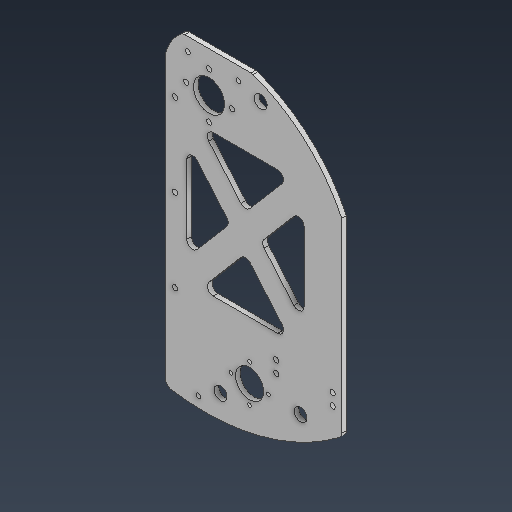
# Autodesk Inventor part: стенка пуляло
Saved by Autodesk Inventor 2026 (Build 300175000, 175)
## iProperties
Created: 2025-11-22
Part Number: стенка пуляло
Material: Типовые
Document SubType Name: Modeling
Designer: Phantom
Density: 1 g/cm^3
Appearance: По умолчанию
Author: Phantom
Autodesk Inventor part; units mm, degrees
(part 1 of 2)
ref_plane "YZ Plane" through (0, 0, 0) normal (1, 0, 0) x (0, 1, 0)
ref_plane "XZ Plane" through (0, 0, 0) normal (0, 1, 0) x (-1, 0, 0)
ref_plane "XY Plane" through (0, 0, 0) normal (0, 0, 1) x (1, 0, 0)
sketch "Эскиз1" plane through (0, 0, 0) normal (0, 0, 1) x (1, 0, 0)
  line L0 (0, 0) -> (150, 0)
  line L1 (150, 0) -> (150, 380)
  line L2 (150, 380) -> (0, 380)
  line L3 (0, 380) -> (0, 0)
  dimension "d2" = 150
  dimension "d3" = 380
  constraints: 8 end point, 2 parallel, 1 horizontal, 1 perpendicular
  measures "d2" distance of L1.end L2.end
  measures "d3" distance of L2.end L0.start
extrude "Выдавливание1" add sketch "Эскиз1" along normal blind 4
sketch "Эскиз3" plane through (0, 0, 0) normal (0, 0, -1) x (-1, 0, 0)
  circle A0 centre (-37, 259.345) radius 3.25
  line L0 (-150, 380) -> (0, 380) projected
  line L1 (0, 380) -> (0, 0) projected
  circle A1 centre (-37, 259.345) radius 203.5
  circle A2 centre (-71.5472, 58.7989) radius 12
  circle A3 centre (-63.3281, 72.5265) radius 1.6
  circle A4 centre (-55.5492, 58.5447) radius 1.6
  circle A5 centre (-63.7683, 44.8172) radius 1.6
  circle A6 centre (-79.7662, 45.0713) radius 1.6
  circle A7 centre (-87.5451, 59.053) radius 1.6
  circle A8 centre (-79.3261, 72.7806) radius 1.6
  line L2 (-162.8639, 128.9118) -> (-165.6991, 126.0733) projected
  arc A9 (-165.6991, 126.0733) -> (-166.6166, 122.0185) centre (-139.5582, 118.0273) ccw projected
  arc A10 (-166.6166, 122.0185) -> (-165.4337, 121.2858) centre (-47.0897, 313.6766) ccw projected
  arc A11 (-165.4337, 121.2858) -> (-162.2121, 123.9136) centre (-181.0608, 143.7331) ccw projected
  arc A12 (-162.2121, 123.9136) -> (-161.041, 123.208) centre (-47.0897, 313.6766) ccw projected
  arc A13 (-161.041, 123.208) -> (-161.8583, 119.1318) centre (-134.7098, 115.8085) ccw projected
  arc A14 (-161.8583, 119.1318) -> (-160.6577, 118.4286) centre (-47.0897, 313.6766) ccw projected
  arc A15 (-160.6577, 118.4286) -> (-157.5019, 121.1349) centre (-176.8332, 140.484) ccw projected
  arc A16 (-157.5019, 121.1349) -> (-156.3138, 120.4584) centre (-47.0897, 313.6766) ccw projected
  arc A17 (-156.3138, 120.4584) -> (-157.0304, 116.3633) centre (-129.8082, 113.7098) ccw projected
  arc A18 (-157.0304, 116.3633) -> (-155.8129, 115.6898) centre (-47.0897, 313.6766) ccw projected
  arc A19 (-155.8129, 115.6898) -> (-152.7247, 118.473) centre (-172.5268, 137.34) ccw projected
  arc A20 (-152.7247, 118.473) -> (-151.5202, 117.826) centre (-47.0897, 313.6766) ccw projected
  arc A21 (-151.5202, 117.826) -> (-152.1357, 113.7145) centre (-124.8564, 111.7326) ccw projected
  arc A22 (-152.1357, 113.7145) -> (-150.902, 113.0712) centre (-47.0897, 313.6766) ccw projected
  arc A23 (-150.902, 113.0712) -> (-147.8833, 115.9297) centre (-168.1442, 134.3031) ccw projected
  arc A24 (-147.8833, 115.9297) -> (-146.6632, 115.3126) centre (-47.0897, 313.6766) ccw projected
  arc A25 (-146.6632, 115.3126) -> (-147.1773, 111.1871) centre (-119.8574, 109.8779) ccw projected
  arc A26 (-147.1773, 111.1871) -> (-145.928, 110.5745) centre (-47.0897, 313.6766) ccw projected
  arc A27 (-145.928, 110.5745) -> (-142.9807, 113.5064) centre (-163.6882, 131.375) ccw projected
  arc A28 (-142.9807, 113.5064) -> (-141.7458, 112.9195) centre (-47.0897, 313.6766) ccw projected
  arc A29 (-141.7458, 112.9195) -> (-142.1581, 108.7827) centre (-114.8143, 108.1469) ccw projected
  arc A30 (-142.1581, 108.7827) -> (-140.8941, 108.201) centre (-47.0897, 313.6766) ccw projected
  arc A31 (-140.8941, 108.201) -> (-138.0199, 111.2047) centre (-159.1613, 128.5577) ccw projected
  arc A32 (-138.0199, 111.2047) -> (-136.771, 110.6484) centre (-47.0897, 313.6766) ccw projected
  arc A33 (-136.771, 110.6484) -> (-137.0811, 106.5027) centre (-109.73, 106.5408) ccw projected
  arc A34 (-137.0811, 106.5027) -> (-135.8033, 105.9522) centre (-47.0897, 313.6766) ccw projected
  arc A35 (-135.8033, 105.9522) -> (-133.0039, 109.0259) centre (-154.5665, 125.8527) ccw projected
  arc A36 (-133.0039, 109.0259) -> (-131.7416, 108.5005) centre (-47.0897, 313.6766) ccw projected
  arc A37 (-131.7416, 108.5005) -> (-131.9496, 104.3484) centre (-104.6077, 105.0603) ccw projected
  arc A38 (-131.9496, 104.3484) -> (-130.6585, 103.8296) centre (-47.0897, 313.6766) ccw projected
  arc A39 (-130.6585, 103.8296) -> (-127.9358, 106.9713) centre (-149.9063, 123.2618) ccw projected
  arc A40 (-127.9358, 106.9713) -> (-126.6609, 106.4772) centre (-47.0897, 313.6766) ccw projected
  arc A41 (-126.6609, 106.4772) -> (-126.7665, 102.3212) centre (-99.4504, 103.7066) ccw projected
  arc A42 (-126.7665, 102.3212) -> (-125.4631, 101.8344) centre (-47.0897, 313.6766) ccw projected
  arc A43 (-125.4631, 101.8344) -> (-122.8185, 105.0422) centre (-145.1838, 120.7864) ccw projected
  arc A44 (-122.8185, 105.0422) -> (-121.5319, 104.5796) centre (-47.0897, 313.6766) ccw projected
  arc A45 (-121.5319, 104.5796) -> (-121.5351, 100.4223) centre (-94.2614, 102.4803) ccw projected
  arc A46 (-121.5351, 100.4223) -> (-120.22, 99.9678) centre (-47.0897, 313.6766) ccw projected
  arc A47 (-120.22, 99.9678) -> (-117.6553, 103.2397) centre (-140.4017, 118.4282) ccw projected
  arc A48 (-117.6553, 103.2397) -> (-116.3577, 102.8091) centre (-47.0897, 313.6766) ccw projected
  arc A49 (-116.3577, 102.8091) -> (-116.2584, 98.6529) centre (-89.0438, 101.3822) ccw projected
  arc A50 (-116.2584, 98.6529) -> (-114.9326, 98.2309) centre (-47.0897, 313.6766) ccw projected
  arc A51 (-114.9326, 98.2309) -> (-112.4493, 101.5651) centre (-135.5629, 116.1885) ccw projected
  arc A52 (-112.4493, 101.5651) -> (-111.1414, 101.1665) centre (-47.0897, 313.6766) ccw projected
  arc A53 (-111.1414, 101.1665) -> (-110.9398, 97.014) centre (-83.8006, 100.413) ccw projected
  arc A54 (-110.9398, 97.014) -> (-109.604, 96.6248) centre (-47.0897, 313.6766) ccw projected
  arc A55 (-109.604, 96.6248) -> (-107.2035, 100.0192) centre (-130.6705, 114.0687) ccw projected
  arc A56 (-107.2035, 100.0192) -> (-105.8863, 99.6529) centre (-47.0897, 313.6766) ccw projected
  arc A57 (-105.8863, 99.6529) -> (-105.5824, 95.5067) centre (-78.5352, 99.5733) ccw projected
  arc A58 (-105.5824, 95.5067) -> (-104.2374, 95.1505) centre (-47.0897, 313.6766) ccw projected
  arc A59 (-104.2374, 95.1505) -> (-101.9213, 98.603) centre (-125.7273, 112.0701) ccw projected
  arc A60 (-101.9213, 98.603) -> (-100.5954, 98.2693) centre (-47.0897, 313.6766) ccw projected
  arc A61 (-100.5954, 98.2693) -> (-100.1895, 94.1318) centre (-73.2507, 98.8635) ccw projected
  arc A62 (-100.1895, 94.1318) -> (-98.8361, 93.8089) centre (-47.0897, 313.6766) ccw projected
  arc A63 (-98.8361, 93.8089) -> (-96.6058, 97.3173) centre (-120.7363, 110.1938) ccw projected
  arc A64 (-96.6058, 97.3173) -> (-95.2721, 97.0164) centre (-47.0897, 313.6766) ccw projected
  arc A65 (-95.2721, 97.0164) -> (-94.7644, 92.8902) centre (-67.9503, 98.2842) ccw projected
  arc A66 (-94.7644, 92.8902) -> (-93.4034, 92.6007) centre (-47.0897, 313.6766) ccw projected
  arc A67 (-93.4034, 92.6007) -> (-91.2602, 96.1631) centre (-115.7007, 108.4411) ccw projected
  arc A68 (-91.2602, 96.1631) -> (-89.9195, 95.8951) centre (-47.0897, 313.6766) ccw projected
  arc A69 (-89.9195, 95.8951) -> (-89.3103, 91.7826) centre (-62.6373, 97.8356) ccw projected
  arc A70 (-89.3103, 91.7826) -> (-88.2236, 91.5786) centre (-47.0897, 313.6766) ccw projected
  line L3 (-88.2236, 91.5786) -> (-86.0083, 96.7219) projected
  line L4 (-86.0083, 96.7219) -> (-85.0766, 98.9705) projected
  arc A71 (-162.8639, 128.9118) -> (-85.0766, 98.9705) centre (-47.0897, 313.6766) ccw projected
  circle A72 centre (-47.0897, 313.6766) radius 225.875
  line L5 (-145.5079, 77.1409) -> (-145.5079, 75.5909) projected
  arc A73 (-145.5079, 75.5909) -> (-144.0079, 74.0909) centre (-144.0079, 75.5909) ccw projected
  line L6 (-144.0079, 74.0909) -> (-92.7079, 74.0909) projected
  arc A74 (-92.7079, 74.0909) -> (-91.2079, 75.5909) centre (-92.7079, 75.5909) ccw projected
  line L7 (-91.2079, 75.5909) -> (-91.2079, 77.1409) projected
  line L8 (-91.2079, 77.1409) -> (-93.3271, 77.1409) projected
  arc A75 (-93.3271, 81.1409) -> (-93.3271, 77.1409) centre (-94.3579, 79.1409) ccw projected
  line L9 (-93.3271, 81.1409) -> (-91.2079, 81.1409) projected
  line L10 (-91.2079, 81.1409) -> (-91.2079, 87.0409) projected
  line L11 (-91.2079, 87.0409) -> (-93.3271, 87.0409) projected
  arc A76 (-93.3271, 91.0409) -> (-93.3271, 87.0409) centre (-94.3579, 89.0409) ccw projected
  line L12 (-93.3271, 91.0409) -> (-91.2079, 91.0409) projected
  line L13 (-91.2079, 91.0409) -> (-91.2079, 92.5909) projected
  arc A77 (-91.2079, 92.5909) -> (-92.7079, 94.0909) centre (-92.7079, 92.5909) ccw projected
  line L14 (-92.7079, 94.0909) -> (-144.0079, 94.0909) projected
  arc A78 (-144.0079, 94.0909) -> (-145.5079, 92.5909) centre (-144.0079, 92.5909) ccw projected
  line L15 (-145.5079, 92.5909) -> (-145.5079, 91.0409) projected
  line L16 (-145.5079, 91.0409) -> (-143.3887, 91.0409) projected
  arc A79 (-143.3887, 87.0409) -> (-143.3887, 91.0409) centre (-142.3579, 89.0409) ccw projected
  line L17 (-143.3887, 87.0409) -> (-145.5079, 87.0409) projected
  line L18 (-145.5079, 87.0409) -> (-145.5079, 81.1409) projected
  line L19 (-145.5079, 81.1409) -> (-143.3887, 81.1409) projected
  arc A80 (-143.3887, 77.1409) -> (-143.3887, 81.1409) centre (-142.3579, 79.1409) ccw projected
  line L20 (-143.3887, 77.1409) -> (-145.5079, 77.1409) projected
  line L21 (-99.5079, 94.0709) -> (-137.8079, 94.0709) projected
  arc A81 (-98.5279, 93.0909) -> (-99.5079, 94.0709) centre (-99.5079, 93.0909) ccw projected
  line L22 (-98.5279, 75.0909) -> (-98.5279, 93.0909) projected
  arc A82 (-99.5079, 74.1109) -> (-98.5279, 75.0909) centre (-99.5079, 75.0909) ccw projected
  line L23 (-137.8079, 74.1109) -> (-99.5079, 74.1109) projected
  arc A83 (-138.7879, 75.0909) -> (-137.8079, 74.1109) centre (-137.8079, 75.0909) ccw projected
  line L24 (-138.7879, 93.0909) -> (-138.7879, 75.0909) projected
  arc A84 (-137.8079, 94.0709) -> (-138.7879, 93.0909) centre (-137.8079, 93.0909) ccw projected
  circle A85 centre (-142.3579, 79.1409) radius 2.25
  circle A86 centre (-142.3579, 89.0409) radius 2.25
  circle A87 centre (-94.3579, 79.1409) radius 2.25
  circle A88 centre (-94.3579, 89.0409) radius 2.25
  circle A89 centre (-37, 259.345) radius 13.25
  line L25 (-37, 259.345) -> (-37, 239.745)
  line L26 (-37, 239.745) -> (-37, 278.945)
  circle A90 centre (-37, 239.745) radius 2.1
  circle A91 centre (-37, 278.945) radius 2.1
  point P0 (-71.5472, 58.7989)
  dimension "d7" = 407
  dimension "d4" = 6.5
  dimension "d5" = 120.655
  dimension "d6" = 37
  dimension "d10" = 26.5
  dimension "d11" = 19.6
  dimension "d12" = 39.2
  dimension "d13" = 4.2
  dimension "d14" = 4.2
  constraints: 15 centre point, 9 coincident, 4 concentric, 4 end point, 1 point on line, 1 vertical, 6 other
  measures "d4" diameter of A0
  measures "d5" distance from line of L0 A0.centre
  measures "d6" distance from line of L1 A0.centre
  measures "d10" diameter of A89
  measures "d11" distance of L25.start L25.end
  measures "d12" distance of L25.end L26.end
  measures "d13" diameter of A90
  measures "d14" diameter of A91
extrude "Выдавливание2" cut sketch "Эскиз3" against normal blind 10 contours A0 L25 L26 | L26 L25 A0 | A2 A1 | A1 A2 | A88 A76 | A86 A79 | A80 A85 | A75 A87 | A3 | A4 | A5 | A6 | A7 | A8
sketch "Эскиз4" plane through (0, 0, 0) normal (0, 0, -1) x (-1, 0, 0)
  circle A0 centre (-37, 259.345) radius 13.25 projected
  circle A1 centre (-37, 278.945) radius 2.1 projected
  circle A2 centre (-37, 239.745) radius 2.1 projected
  point P0 (0, 0)
extrude "Выдавливание3" cut sketch "Эскиз3" against normal blind 10 contours A0 L25 L26 | A0 L26 A89 L25 | L26 L25 A0 | A0 L25 A89 L26 | A90 | A91
sketch "Эскиз5" plane through (150, 0, 0) normal (1, 0, 0) x (0, 0, -1)
  line L0 (-4, 380) -> (-4, 0) projected
  line L1 (-4, 30) -> (0, 30)
  line L2 (0, 0) -> (-4, 0) projected
  line L3 (-4, 290) -> (0, 290)
  line L4 (0, 0) -> (0, 380) projected
  line L5 (0, 380) -> (-4, 380) projected
  dimension "d17" = 30
  dimension "d18" = 90
  constraints: 4 end point, 3 point on line, 1 horizontal, 1 perpendicular
  measures "d17" distance between parallel lines of L2 L1
  measures "d18" distance between parallel lines of L3 L5
extrude "Выдавливание4" cut sketch "Эскиз5" against normal through all contours L5 L4 L3 L0 | L1 L4 L2 L0
sketch "Эскиз6" plane through (0, 0, 0) normal (0, 0, -1) x (-1, 0, 0)
  circle A0 centre (-37, 259.345) radius 13.25 projected
  circle A1 centre (-37, 259.345) radius 229.345
  line L0 (0, 30) -> (-150, 30) projected
  circle A2 centre (-37, 259.345) radius 37.9855
  line L1 (-150, 30) -> (-150, 290) projected
  arc A3 (-40.2154, 297.1942) -> (-150, 221.3595) centre (-28.8449, 163.3493) ccw
  circle A4 centre (-142.3579, 89.0409) radius 2.25 projected
  circle A5 centre (-79.3261, 72.7806) radius 1.6 projected
  circle A6 centre (-63.7683, 44.8172) radius 1.6 projected
  circle A7 centre (-79.7662, 45.0713) radius 1.6 projected
  circle A8 centre (-94.3579, 79.1409) radius 2.25 projected
  circle A9 centre (-142.3579, 79.1409) radius 2.25 projected
  circle A10 centre (-71.5472, 58.7989) radius 12 projected
  circle A11 centre (-63.3281, 72.5265) radius 1.6 projected
  circle A12 centre (-55.5492, 58.5447) radius 1.6 projected
  circle A13 centre (-87.5451, 59.053) radius 1.6 projected
  circle A14 centre (-94.3579, 89.0409) radius 2.25 projected
  circle A15 centre (-37, 259.345) radius 13.25 projected
  circle A16 centre (-37, 278.945) radius 2.1 projected
  circle A17 centre (-37, 239.745) radius 2.1 projected
  line L2 (0, 290) -> (-150, 290) projected
  line L3 (-150, 30) -> (-150, 290) projected
  line L4 (-150, 30) -> (0, 30) projected
  line L5 (0, 290) -> (0, 30) projected
  point P0 (0, 0)
  point P1 (0, 267.9415)
  point P2 (-14.5685, 290)
  point P3 (-73.6036, 290)
  point P4 (0, 33.0043)
  point P5 (-37, 30)
  point P6 (-150, 59.7701)
  constraints: 2 centre point, 2 coincident, 2 point on circle, 1 point on line, 1 tangent, 4 other
extrude "Выдавливание5" cut sketch "Эскиз6" against normal blind 10 contours A1 L0 L1 | L5 L0 A1 | L1 L2 A3 | A2 L2 L5 picked at (-4.9355, 285.277)
fillet "Сопряжение1" radius 5 4 edges at (73.6036, 290, 2) (14.5685, 290, 2) (150, 59.7701, 2) (0, 33.0043, 2)
sketch "Эскиз7" plane through (0, 0, 0) normal (0, 0, -1) x (-1, 0, 0)
  circle A0 centre (-37, 259.345) radius 35 projected
  circle A1 centre (-81, 273) radius 5.5
  line L0 (-16.2668, 290) -> (-72.7377, 290) projected
  circle A2 centre (-115, 59.0909) radius 5.5
  line L1 (-150, 62.7066) -> (-150, 221.3595) projected
  line L2 (-144.0079, 74.0909) -> (-92.7079, 74.0909) projected
  point P0 (0, 0)
  dimension "d24" = 11
  dimension "d25" = 17
  dimension "d26" = 44
  dimension "d27" = 11
  dimension "d28" = 35
  dimension "d29" = 15
  constraints: 2 centre point
  measures "d24" diameter of A1
  measures "d25" distance from line of A1.centre L0
  measures "d26" horizontal distance of A0.centre A1.centre
  measures "d27" diameter of A2
  measures "d28" distance from line of A2.centre L1
  measures "d29" distance from line of A2.centre L2
extrude "Выдавливание6" cut sketch "Эскиз7" against normal blind 10 contours A1 | A2
sketch "Эскиз8" plane through (0, 0, 0) normal (0, 0, -1) x (-1, 0, 0)
  line L0 (0, 167.3772) -> (0, 171.6772) projected
  line L1 (0, 169.5272) -> (-8, 169.5272)
  line L2 (0, 97.0611) -> (0, 101.3611) projected
  line L3 (0, 237.7901) -> (0, 242.0901) projected
  line L4 (0, 239.9401) -> (-8, 239.9401)
  line L5 (0, 99.2111) -> (-8, 99.2111)
  circle A0 centre (-8, 99.2111) radius 2.25
  circle A1 centre (-8, 169.5272) radius 2.25
  circle A2 centre (-8, 239.9401) radius 2.25
  point P0 (0, 0)
  dimension "d32" = 8
  dimension "d33" = 4.5
  dimension "d34" = 8
  dimension "d35" = 8
  constraints: 6 end point, 3 centre point, 3 coincident, 3 horizontal, 3 midpoint
  measures "d32" distance of L5.start L5.end
  measures "d33" diameter of A0
  measures "d34" distance of L1.start L1.end
  measures "d35" distance of L4.start L4.end
extrude "Выдавливание7" cut sketch "Эскиз8" against normal blind 10
sketch "Эскиз9" plane through (0, 0, 0) normal (0, 0, -1) x (-1, 0, 0)
  point P0 (0, 0)
sketch "Эскиз10" plane through (0, 0, 0) normal (0, 0, -1) x (-1, 0, 0)
  arc A0 (-13.7181, 39.7264) -> (-18.4467, 38.1012) centre (-22.0897, 56.392) ccw projected
  arc A1 (-53.1661, 61.9546) -> (-52.9883, 56.9578) centre (-71.5472, 58.7989) ccw projected
  circle A2 centre (-62, 278.7903) radius 2.1
  circle A3 centre (-19, 278.7903) radius 2.1
  circle A4 centre (-37, 278.945) radius 2.1 projected
  circle A5 centre (-46.8597, 40.7124) radius 5.5
  line L0 (-52.9883, 56.9578) -> (-40.7311, 56.9578)
  line L1 (-46.8597, 56.9578) -> (-46.8597, 30.5679)
  point P0 (0, 0)
  dimension "d38" = 4.2
  dimension "d39" = 4.2
  dimension "d40" = 18
  dimension "d41" = 25
  dimension "d42" = 11
  dimension "d43" = 0
  constraints: 4 end point, 3 centre point, 1 horizontal, 1 midpoint, 1 point on circle, 1 vertical
  measures "d38" diameter of A2
  measures "d39" diameter of A3
  measures "d40" horizontal distance of A4.centre A3.centre
  measures "d41" horizontal distance of A4.centre A2.centre
  measures "d42" diameter of A5
  measures "d43" distance from line of L1 A5.centre
extrude "Выдавливание8" cut sketch "Эскиз10" against normal blind 10 contours A2 | A3 | A5 L1 | L1 A5
sketch "Эскиз11" plane through (0, 0, 0) normal (0, 0, -1) x (-1, 0, 0)
  line L0 (-0.9763, 60.1051) -> (-14.0486, 76.2641) projected
  arc A0 (-14.0486, 76.2641) -> (-14.7486, 76.5333) centre (-14.6317, 75.7924) ccw projected
  line L1 (-14.7486, 76.5333) -> (-35.2789, 73.2919) projected
  arc A1 (-35.2789, 73.2919) -> (-35.862, 72.8202) centre (-35.162, 72.551) ccw projected
  line L2 (-35.862, 72.8202) -> (-43.32, 53.4197) projected
  arc A2 (-43.32, 53.4197) -> (-43.2031, 52.6789) centre (-42.62, 53.1506) ccw projected
  line L3 (-43.2031, 52.6789) -> (-30.1308, 36.5198) projected
  arc A3 (-30.1308, 36.5198) -> (-29.4308, 36.2507) centre (-29.5477, 36.9915) ccw projected
  line L4 (-29.4308, 36.2507) -> (-8.9004, 39.4921) projected
  arc A4 (-8.9004, 39.4921) -> (-8.3174, 39.9638) centre (-9.0174, 40.2329) ccw projected
  line L5 (-8.3174, 39.9638) -> (-0.8593, 59.3642) projected
  arc A5 (-0.8593, 59.3642) -> (-0.9763, 60.1051) centre (-1.5594, 59.6334) ccw projected
  arc A6 (-8.4897, 56.8181) -> (-9.02, 60.1765) centre (-8.7549, 58.4973) ccw projected
  line L6 (-8.4897, 56.8181) -> (-10.0702, 56.5686) projected
  arc A7 (-10.6004, 59.927) -> (-10.0702, 56.5686) centre (-10.3353, 58.2478) ccw projected
  line L7 (-9.02, 60.1765) -> (-10.6004, 59.927) projected
  line L8 (-33.579, 52.857) -> (-35.1594, 52.6074) projected
  arc A8 (-35.6896, 55.9658) -> (-35.1594, 52.6074) centre (-35.4245, 54.2866) ccw projected
  line L9 (-34.1092, 56.2154) -> (-35.6896, 55.9658) projected
  arc A9 (-33.579, 52.857) -> (-34.1092, 56.2154) centre (-33.8441, 54.5362) ccw projected
  circle A10 centre (-33.7095, 70.7556) radius 1.25 projected
  circle A11 centre (-3.8405, 59.2732) radius 1.25 projected
  circle A12 centre (-28.719, 39.1471) radius 1.25 projected
  circle A13 centre (-40.3388, 53.5107) radius 1.25 projected
  circle A14 centre (-15.4603, 73.6368) radius 1.25 projected
  circle A15 centre (-10.4699, 42.0283) radius 1.25 projected
  circle A16 centre (-22.0897, 56.392) radius 6.5 projected
  circle A17 centre (-62, 278.7903) radius 2.1 projected
  circle A18 centre (-19, 278.7903) radius 2.1 projected
  circle A19 centre (-46.8597, 40.7124) radius 5.5 projected
  circle A20 centre (-8, 239.9401) radius 2.25 projected
  circle A21 centre (-8, 169.5272) radius 2.25 projected
  circle A22 centre (-8, 99.2111) radius 2.25 projected
  circle A23 centre (-81, 273) radius 5.5 projected
  circle A24 centre (-115, 59.0909) radius 5.5 projected
  circle A25 centre (-37, 239.745) radius 2.1 projected
  circle A26 centre (-37, 278.945) radius 2.1 projected
  circle A27 centre (-37, 259.345) radius 13.25 projected
  circle A28 centre (-94.3579, 89.0409) radius 2.25 projected
  circle A29 centre (-87.5451, 59.053) radius 1.6 projected
  circle A30 centre (-55.5492, 58.5447) radius 1.6 projected
  circle A31 centre (-63.3281, 72.5265) radius 1.6 projected
  circle A32 centre (-71.5472, 58.7989) radius 12 projected
  circle A33 centre (-142.3579, 79.1409) radius 2.25 projected
  circle A34 centre (-94.3579, 79.1409) radius 2.25 projected
  circle A35 centre (-79.7662, 45.0713) radius 1.6 projected
  circle A36 centre (-63.7683, 44.8172) radius 1.6 projected
  circle A37 centre (-79.3261, 72.7806) radius 1.6 projected
  circle A38 centre (-142.3579, 89.0409) radius 2.25 projected
  arc A39 (-4.2868, 32.3451) -> (0, 37.2939) centre (-5, 37.2939) ccw projected
  line L10 (0, 267.9415) -> (0, 37.2939) projected
  arc A40 (0, 267.9415) -> (-13.124, 288.8888) centre (-37, 259.345) ccw projected
  arc A41 (-13.124, 288.8888) -> (-16.2668, 290) centre (-16.2668, 285) ccw projected
  line L11 (-16.2668, 290) -> (-72.7377, 290) projected
  arc A42 (-72.7377, 290) -> (-74.4347, 289.7032) centre (-72.7377, 285) ccw projected
  arc A43 (-74.4347, 289.7032) -> (-150, 221.3595) centre (-28.8449, 163.3493) ccw projected
  line L12 (-150, 62.7066) -> (-150, 221.3595) projected
  arc A44 (-150, 62.7066) -> (-147.407, 58.3241) centre (-145, 62.7066) ccw projected
  arc A45 (-147.407, 58.3241) -> (-4.2868, 32.3451) centre (-37, 259.345) ccw projected
  arc A46 (-2.8604, 22.4473) -> (10, 37.2939) centre (-5, 37.2939) ccw
  arc A47 (-152.221, 49.559) -> (-2.8604, 22.4473) centre (-37, 259.345) ccw
  arc A48 (-160, 62.7066) -> (-152.221, 49.559) centre (-145, 62.7066) ccw
  line L13 (-160, 62.7066) -> (-160, 223.5873)
  arc A49 (-77.8286, 299.1097) -> (-160, 223.5873) centre (-28.8449, 163.3493) ccw
  arc A50 (-72.7377, 300) -> (-77.8286, 299.1097) centre (-72.7377, 285) ccw
  line L14 (-72.7377, 300) -> (-16.2668, 300)
  arc A51 (-6.8385, 296.6665) -> (-16.2668, 300) centre (-16.2668, 285) ccw
  arc A52 (10, 269.0202) -> (-6.8385, 296.6665) centre (-37, 259.345) ccw
  line L15 (10, 269.0202) -> (10, 37.2939)
  circle A53 centre (-5.75, 29.2915) radius 2.1
  circle A54 centre (-27.8653, 29.2915) radius 2.1
  line L16 (-27.8653, 29.2915) -> (-5.75, 29.2915)
  line L17 (-16.2668, 290) -> (-72.7377, 290) projected
  line L18 (0, 37.2939) -> (0, 23.1518)
  line L19 (-150, 62.7066) -> (-150, 48.3544)
  arc A55 (-147.407, 58.3241) -> (0, 23.1518) centre (-33.7733, 208.0855) ccw
  point P0 (0, 0)
  point P1 (-29.8168, 36.2915)
  point P2 (-29.7979, 30.1131)
  point P3 (-25.7653, 20.2638)
  point P4 (-18.1652, 20.7422)
  point P5 (-26.0039, 30.2638)
  point P6 (-14.7486, -223.0943)
  point P7 (-35.862, -219.3812)
  point P8 (-43.2031, -199.2399)
  point P9 (-29.4308, -182.8117)
  point P10 (-8.3174, -186.5248)
  dimension "d46" = 10
  dimension "d47" = 4.2
  dimension "d48" = 4.2
  dimension "d49" = 7
  constraints: 19 point on circle, 12 end point, 10 centre point, 2 parallel, 1 vertical, 9 other
  measures "d46" radial gap between concentric circles of A39 A46
  measures "d47" diameter of A53
  measures "d48" diameter of A54
  measures "d49" distance from line of point (-29.817, 36.291) L16
extrude "Выдавливание9" add sketch "Эскиз11" against normal up to surface (4 mm away) contours A39 L18 A55 A47 A45 A54 | A54 A45 | A55 A47 | A53 picked at (-27.7819, 29.193)
sketch "Эскиз12" plane through (0, 0, 0) normal (0, 0, -1) x (-1, 0, 0)
  arc A0 (-29.7979, 30.1131) -> (-26.0039, 30.2638) centre (-27.8653, 29.2915) ccw projected
  circle A1 centre (-27.8653, 29.2915) radius 2.1
  point P0 (0, 0)
  point P1 (-29.7979, 30.1131)
  constraints: 1 centre point, 1 coincident
extrude "Выдавливание10" cut sketch "Эскиз12" against normal blind 10
fillet "Сопряжение2" radius 5 2 edges at (0, 23.1518, 2) (147.407, 58.3241, 2)
sketch "Эскиз13" plane through (0, 0, 0) normal (0, 0, -1) x (-1, 0, 0)
  arc A0 (-4.2138, 22.4317) -> (0, 27.3695) centre (-5, 27.3695) ccw projected
  line L0 (0, 267.9415) -> (0, 27.3695) projected
  arc A1 (0, 267.9415) -> (-13.124, 288.8888) centre (-37, 259.345) ccw projected
  arc A2 (-13.124, 288.8888) -> (-16.2668, 290) centre (-16.2668, 285) ccw projected
  line L1 (-16.2668, 290) -> (-72.7377, 290) projected
  arc A3 (-72.7377, 290) -> (-74.4347, 289.7032) centre (-72.7377, 285) ccw projected
  arc A4 (-74.4347, 289.7032) -> (-150, 221.3595) centre (-28.8449, 163.3493) ccw projected
  line L2 (-150, 62.7066) -> (-150, 221.3595) projected
  arc A5 (-150, 62.7066) -> (-147.5924, 58.4311) centre (-145, 62.7066) ccw projected
  arc A6 (-147.1688, 58.1436) -> (-147.5924, 58.4311) centre (-150.1848, 54.1556) ccw projected
  arc A7 (-147.1688, 58.1436) -> (-4.2138, 22.4317) centre (-33.7733, 208.0855) ccw projected
  circle A8 centre (-62, 278.7903) radius 2.1 projected
  circle A9 centre (-19, 278.7903) radius 2.1 projected
  circle A10 centre (-46.8597, 40.7124) radius 5.5 projected
  circle A11 centre (-8, 239.9401) radius 2.25 projected
  circle A12 centre (-8, 169.5272) radius 2.25 projected
  circle A13 centre (-8, 99.2111) radius 2.25 projected
  circle A14 centre (-81, 273) radius 5.5 projected
  circle A15 centre (-115, 59.0909) radius 5.5 projected
  circle A16 centre (-37, 239.745) radius 2.1 projected
  circle A17 centre (-37, 278.945) radius 2.1 projected
  circle A18 centre (-37, 259.345) radius 13.25 projected
  circle A19 centre (-94.3579, 89.0409) radius 2.25 projected
  circle A20 centre (-87.5451, 59.053) radius 1.6 projected
  circle A21 centre (-55.5492, 58.5447) radius 1.6 projected
  circle A22 centre (-63.3281, 72.5265) radius 1.6 projected
  circle A23 centre (-71.5472, 58.7989) radius 12 projected
  circle A24 centre (-142.3579, 79.1409) radius 2.25 projected
  circle A25 centre (-94.3579, 79.1409) radius 2.25 projected
  circle A26 centre (-79.7662, 45.0713) radius 1.6 projected
  circle A27 centre (-63.7683, 44.8172) radius 1.6 projected
  circle A28 centre (-79.3261, 72.7806) radius 1.6 projected
  circle A29 centre (-142.3579, 89.0409) radius 2.25 projected
  line L3 (-8, 99.2111) -> (-128, 99.2111)
  line L4 (-128, 99.2111) -> (-128, 239.9401)
  line L5 (-128, 239.9401) -> (-8, 239.9401)
  line L6 (-8, 239.9401) -> (-8, 99.2111)
  line L7 (-128, 99.2111) -> (-8, 239.9401)
  line L8 (-128, 239.9401) -> (-8, 99.2111)
  line L9 (-120.3908, 92.7227) -> (-0.3908, 233.4517)
  line L10 (-135.6092, 105.6995) -> (-15.6092, 246.4285)
  line L11 (-135.6092, 233.4517) -> (-15.6092, 92.7227)
  line L12 (-120.3908, 246.4285) -> (-0.3908, 105.6995)
  line L13 (-18, 99.2111) -> (-18, 239.9401)
  line L14 (-128, 229.9401) -> (-18, 229.9401)
  line L15 (-18, 229.9401) -> (-18, 99.2111)
  line L16 (-118, 99.2111) -> (-118, 239.9401)
  line L17 (-8, 109.2111) -> (-128, 109.2111)
  point P0 (-81.1419, 169.5756)
  point P1 (-128, 224.528)
  point P2 (-128, 114.6232)
  point P3 (-29.6689, 229.9401)
  point P4 (-106.3311, 229.9401)
  point P5 (-68, 184.9877)
  point P6 (-18, 126.3506)
  point P7 (-18, 212.8006)
  point P8 (-54.8581, 169.5756)
  point P9 (-21.1419, 99.2111)
  point P10 (-68, 154.1635)
  point P11 (-114.8581, 99.2111)
  point P12 (-118, 212.8006)
  point P13 (-118, 126.3506)
  point P14 (-106.3311, 109.2111)
  point P15 (-29.6689, 109.2111)
  dimension "d57" = 0
  dimension "d58" = 120
  dimension "d59" = 10
  dimension "d60" = 10
  dimension "d61" = 10
  dimension "d62" = 10
  dimension "d63" = 10
  dimension "d64" = 10
  dimension "d67" = 10
  dimension "d68" = 10
  constraints: 30 end point, 8 parallel, 1 horizontal, 1 perpendicular, 1 point on line, 1 other
  measures "d57" distance from line of L7.end L5
  measures "d58" distance of L4.end L5.end
  measures "d59" distance between parallel lines of L7 L9
  measures "d60" distance between parallel lines of L7 L10
  measures "d61" distance between parallel lines of L8 L11
  measures "d62" distance between parallel lines of L8 L12
  measures "d63" distance between parallel lines of L6 L13
  measures "d64" distance between parallel lines of L5 L14
  measures "d67" distance between parallel lines of L4 L16
  measures "d68" distance between parallel lines of L3 L17
extrude "Выдавливание11" cut sketch "Эскиз13" against normal blind 10 contours L13 L12 L9 | L10 L12 L14 | L11 L17 L9 | L10 L16 L11
fillet "Сопряжение3" radius 5 12 edges at (29.6689, 229.9401, 2) (29.6689, 109.2111, 2) (18, 126.3506, 2) (18, 212.8006, 2) (54.8581, 169.5756, 2) (68, 154.1635, 2) (106.3311, 109.2111, 2) (81.1419, 169.5756, 2) (68, 184.9877, 2) (106.3311, 229.9401, 2) (118, 212.8006, 2) (118, 126.3506, 2)
sketch "Эскиз14" plane through (0, 0, 0) normal (0, 0, -1) x (-1, 0, 0)
  line L0 (-26.8046, 136.6761) -> (-52.0917, 166.3314) projected
  arc A0 (-52.0917, 172.8198) -> (-52.0917, 166.3314) centre (-48.2871, 169.5756) ccw projected
  line L1 (-52.0917, 172.8198) -> (-26.8046, 202.4751) projected
  arc A1 (-18, 199.2309) -> (-26.8046, 202.4751) centre (-23, 199.2309) ccw projected
  line L2 (-18, 199.2309) -> (-18, 139.9204) projected
  arc A2 (-26.8046, 136.6761) -> (-18, 139.9204) centre (-23, 139.9204) ccw projected
  line L3 (-109.1954, 202.4751) -> (-83.9083, 172.8198) projected
  arc A3 (-83.9083, 166.3314) -> (-83.9083, 172.8198) centre (-87.7129, 169.5756) ccw projected
  line L4 (-83.9083, 166.3314) -> (-109.1954, 136.6761) projected
  arc A4 (-118, 139.9204) -> (-109.1954, 136.6761) centre (-113, 139.9204) ccw projected
  line L5 (-118, 139.9204) -> (-118, 199.2309) projected
  arc A5 (-109.1954, 202.4751) -> (-118, 199.2309) centre (-113, 199.2309) ccw projected
  line L6 (-36.6988, 221.6959) -> (-64.1954, 189.4495) projected
  arc A6 (-71.8046, 189.4495) -> (-64.1954, 189.4495) centre (-68, 192.6937) ccw projected
  line L7 (-71.8046, 189.4495) -> (-99.3012, 221.6959) projected
  arc A7 (-95.4966, 229.9401) -> (-99.3012, 221.6959) centre (-95.4966, 224.9401) ccw projected
  line L8 (-95.4966, 229.9401) -> (-40.5034, 229.9401) projected
  arc A8 (-36.6988, 221.6959) -> (-40.5034, 229.9401) centre (-40.5034, 224.9401) ccw projected
  line L9 (-99.3012, 117.4553) -> (-71.8046, 149.7017) projected
  arc A9 (-64.1954, 149.7017) -> (-71.8046, 149.7017) centre (-68, 146.4575) ccw projected
  line L10 (-64.1954, 149.7017) -> (-36.6988, 117.4553) projected
  arc A10 (-40.5034, 109.2111) -> (-36.6988, 117.4553) centre (-40.5034, 114.2111) ccw projected
  line L11 (-40.5034, 109.2111) -> (-95.4966, 109.2111) projected
  arc A11 (-99.3012, 117.4553) -> (-95.4966, 109.2111) centre (-95.4966, 114.2111) ccw projected
  arc A12 (-4.2138, 22.4317) -> (0, 27.3695) centre (-5, 27.3695) ccw projected
  line L12 (0, 267.9415) -> (0, 27.3695) projected
  arc A13 (0, 267.9415) -> (-13.124, 288.8888) centre (-37, 259.345) ccw projected
  arc A14 (-13.124, 288.8888) -> (-16.2668, 290) centre (-16.2668, 285) ccw projected
  line L13 (-16.2668, 290) -> (-72.7377, 290) projected
  arc A15 (-72.7377, 290) -> (-74.4347, 289.7032) centre (-72.7377, 285) ccw projected
  arc A16 (-74.4347, 289.7032) -> (-150, 221.3595) centre (-28.8449, 163.3493) ccw projected
  line L14 (-150, 62.7066) -> (-150, 221.3595) projected
  arc A17 (-150, 62.7066) -> (-147.5924, 58.4311) centre (-145, 62.7066) ccw projected
  arc A18 (-147.1688, 58.1436) -> (-147.5924, 58.4311) centre (-150.1848, 54.1556) ccw projected
  arc A19 (-147.1688, 58.1436) -> (-4.2138, 22.4317) centre (-33.7733, 208.0855) ccw projected
  circle A20 centre (-62, 278.7903) radius 2.1 projected
  circle A21 centre (-19, 278.7903) radius 2.1 projected
  circle A22 centre (-46.8597, 40.7124) radius 5.5 projected
  circle A23 centre (-8, 239.9401) radius 2.25 projected
  circle A24 centre (-8, 169.5272) radius 2.25 projected
  circle A25 centre (-8, 99.2111) radius 2.25 projected
  circle A26 centre (-81, 273) radius 5.5 projected
  circle A27 centre (-115, 59.0909) radius 5.5 projected
  circle A28 centre (-37, 239.745) radius 2.1 projected
  circle A29 centre (-37, 278.945) radius 2.1 projected
  circle A30 centre (-37, 259.345) radius 13.25 projected
  circle A31 centre (-94.3579, 89.0409) radius 2.25 projected
  circle A32 centre (-87.5451, 59.053) radius 1.6 projected
  circle A33 centre (-55.5492, 58.5447) radius 1.6 projected
  circle A34 centre (-63.3281, 72.5265) radius 1.6 projected
  circle A35 centre (-71.5472, 58.7989) radius 12 projected
  circle A36 centre (-142.3579, 79.1409) radius 2.25 projected
  circle A37 centre (-94.3579, 79.1409) radius 2.25 projected
  circle A38 centre (-79.7662, 45.0713) radius 1.6 projected
  circle A39 centre (-63.7683, 44.8172) radius 1.6 projected
  circle A40 centre (-79.3261, 72.7806) radius 1.6 projected
  circle A41 centre (-142.3579, 89.0409) radius 2.25 projected
  circle A42 centre (-37, 253.345) radius 13.25
  circle A43 centre (-37, 259.345) radius 13.25 projected
  line L15 (-37, 272.595) -> (-37, 266.595)
  line L16 (-56.6, 253.345) -> (-17.4, 253.345)
  circle A44 centre (-56.6, 253.345) radius 2.15
  circle A45 centre (-17.4, 253.345) radius 2.15
  point P0 (0, 0)
  dimension "d71" = 26.5
  dimension "d73" = 39.2
  dimension "d74" = 4.3
  dimension "d75" = 4.3
  constraints: 4 end point, 2 centre point, 2 coincident, 2 vertical alignment, 3 other
  measures "d73" distance of L16.start L16.end
  measures "d74" diameter of A44
  measures "d75" diameter of A45
extrude "Выдавливание12" cut sketch "Эскиз14" against normal blind 10 contours A42 A28 | A28 A42 L16 A30 | L16 A30 A42 | A42 A30 L16 | A30 L16 A42 | A30 L16 | A44 | A45 picked at (-36.9158, 240.6849)
sketch "Эскиз15" plane through (0, 0, 0) normal (0, 0, -1) x (-1, 0, 0)
  arc A0 (-49.9059, 256.345) -> (-39.0377, 240.2526) centre (-37, 253.345) ccw projected
  circle A1 centre (-37, 253.345) radius 13.25
  arc A2 (-34.9623, 240.2526) -> (-24.0941, 256.345) centre (-37, 253.345) ccw projected
  arc A3 (-39.0377, 240.2526) -> (-34.9623, 240.2526) centre (-37, 239.745) ccw projected
  arc A4 (-49.9059, 256.345) -> (-39.0377, 240.2526) centre (-37, 253.345) ccw projected
  arc A5 (-24.0941, 256.345) -> (-49.9059, 256.345) centre (-37, 259.345) ccw projected
  circle A6 centre (-17.4, 253.345) radius 2.15 projected
  circle A7 centre (-56.6, 253.345) radius 2.15 projected
  line L0 (-26.8046, 136.6761) -> (-52.0917, 166.3314) projected
  arc A8 (-52.0917, 172.8198) -> (-52.0917, 166.3314) centre (-48.2871, 169.5756) ccw projected
  line L1 (-52.0917, 172.8198) -> (-26.8046, 202.4751) projected
  arc A9 (-18, 199.2309) -> (-26.8046, 202.4751) centre (-23, 199.2309) ccw projected
  line L2 (-18, 199.2309) -> (-18, 139.9204) projected
  arc A10 (-26.8046, 136.6761) -> (-18, 139.9204) centre (-23, 139.9204) ccw projected
  line L3 (-109.1954, 202.4751) -> (-83.9083, 172.8198) projected
  arc A11 (-83.9083, 166.3314) -> (-83.9083, 172.8198) centre (-87.7129, 169.5756) ccw projected
  line L4 (-83.9083, 166.3314) -> (-109.1954, 136.6761) projected
  arc A12 (-118, 139.9204) -> (-109.1954, 136.6761) centre (-113, 139.9204) ccw projected
  line L5 (-118, 139.9204) -> (-118, 199.2309) projected
  arc A13 (-109.1954, 202.4751) -> (-118, 199.2309) centre (-113, 199.2309) ccw projected
  line L6 (-36.6988, 221.6959) -> (-64.1954, 189.4495) projected
  arc A14 (-71.8046, 189.4495) -> (-64.1954, 189.4495) centre (-68, 192.6937) ccw projected
  line L7 (-71.8046, 189.4495) -> (-99.3012, 221.6959) projected
  arc A15 (-95.4966, 229.9401) -> (-99.3012, 221.6959) centre (-95.4966, 224.9401) ccw projected
  line L8 (-95.4966, 229.9401) -> (-40.5034, 229.9401) projected
  arc A16 (-36.6988, 221.6959) -> (-40.5034, 229.9401) centre (-40.5034, 224.9401) ccw projected
  line L9 (-99.3012, 117.4553) -> (-71.8046, 149.7017) projected
  arc A17 (-64.1954, 149.7017) -> (-71.8046, 149.7017) centre (-68, 146.4575) ccw projected
  line L10 (-64.1954, 149.7017) -> (-36.6988, 117.4553) projected
  arc A18 (-40.5034, 109.2111) -> (-36.6988, 117.4553) centre (-40.5034, 114.2111) ccw projected
  line L11 (-40.5034, 109.2111) -> (-95.4966, 109.2111) projected
  arc A19 (-99.3012, 117.4553) -> (-95.4966, 109.2111) centre (-95.4966, 114.2111) ccw projected
  arc A20 (-4.2138, 22.4317) -> (0, 27.3695) centre (-5, 27.3695) ccw projected
  line L12 (0, 267.9415) -> (0, 27.3695) projected
  arc A21 (0, 267.9415) -> (-13.124, 288.8888) centre (-37, 259.345) ccw projected
  arc A22 (-13.124, 288.8888) -> (-16.2668, 290) centre (-16.2668, 285) ccw projected
  line L13 (-16.2668, 290) -> (-72.7377, 290) projected
  arc A23 (-72.7377, 290) -> (-74.4347, 289.7032) centre (-72.7377, 285) ccw projected
  arc A24 (-74.4347, 289.7032) -> (-150, 221.3595) centre (-28.8449, 163.3493) ccw projected
  line L14 (-150, 62.7066) -> (-150, 221.3595) projected
  arc A25 (-150, 62.7066) -> (-147.5924, 58.4311) centre (-145, 62.7066) ccw projected
  arc A26 (-147.1688, 58.1436) -> (-147.5924, 58.4311) centre (-150.1848, 54.1556) ccw projected
  arc A27 (-147.1688, 58.1436) -> (-4.2138, 22.4317) centre (-33.7733, 208.0855) ccw projected
  circle A28 centre (-62, 278.7903) radius 2.1 projected
  circle A29 centre (-19, 278.7903) radius 2.1 projected
  circle A30 centre (-46.8597, 40.7124) radius 5.5 projected
  circle A31 centre (-8, 239.9401) radius 2.25 projected
  circle A32 centre (-8, 169.5272) radius 2.25 projected
  circle A33 centre (-8, 99.2111) radius 2.25 projected
  circle A34 centre (-81, 273) radius 5.5 projected
  circle A35 centre (-115, 59.0909) radius 5.5 projected
  circle A36 centre (-37, 278.945) radius 2.1 projected
  circle A37 centre (-94.3579, 89.0409) radius 2.25 projected
  circle A38 centre (-87.5451, 59.053) radius 1.6 projected
  circle A39 centre (-55.5492, 58.5447) radius 1.6 projected
  circle A40 centre (-63.3281, 72.5265) radius 1.6 projected
  circle A41 centre (-71.5472, 58.7989) radius 12 projected
  circle A42 centre (-142.3579, 79.1409) radius 2.25 projected
  circle A43 centre (-94.3579, 79.1409) radius 2.25 projected
  circle A44 centre (-79.7662, 45.0713) radius 1.6 projected
  circle A45 centre (-63.7683, 44.8172) radius 1.6 projected
  circle A46 centre (-79.3261, 72.7806) radius 1.6 projected
  circle A47 centre (-142.3579, 89.0409) radius 2.25 projected
  point P0 (0, 0)
  point P1 (-49.9059, 256.345)
  point P2 (-24.0941, 256.345)
  constraints: 1 centre point, 1 coincident, 1 concentric
extrude "Выдавливание13" add sketch "Эскиз15" against normal up to surface (4 mm away) contours A5 A1 | A1 A3 | A36
sketch "Эскиз16" plane through (0, 0, 0) normal (0, 0, -1) x (-1, 0, 0)
  circle A0 centre (-27.8653, 29.2915) radius 2.1 projected
  circle A1 centre (-142.3579, 79.1409) radius 2.25 projected
  circle A2 centre (-142.3579, 89.0409) radius 2.25 projected
  circle A3 centre (-94.3579, 89.0409) radius 2.25 projected
  circle A4 centre (-94.3579, 79.1409) radius 2.25 projected
  line L0 (-89.1248, 59.3072) -> (-89.1248, 66.9978)
  arc A5 (-85.9655, 66.9978) -> (-89.1248, 66.9978) centre (-87.5451, 66.9978) ccw
  line L1 (-85.9655, 66.9978) -> (-85.9655, 59.3072)
  arc A6 (-85.9655, 58.7989) -> (-85.9655, 59.3072) centre (-87.5451, 59.053) ccw
  line L2 (-85.9655, 58.7989) -> (-85.9655, 51.1083)
  arc A7 (-89.1248, 51.1083) -> (-85.9655, 51.1083) centre (-87.5451, 51.1083) ccw
  line L3 (-89.1248, 51.1083) -> (-89.1248, 58.7989)
  arc A8 (-89.1248, 59.3072) -> (-89.1248, 58.7989) centre (-87.5451, 59.053) ccw
  circle A9 centre (-115, 59.0909) radius 5.5 projected
  circle A10 centre (-81, 273) radius 5.5 projected
  circle A11 centre (-8, 99.2111) radius 2.25 projected
  circle A12 centre (-8, 169.5272) radius 2.25 projected
  circle A13 centre (-8, 239.9401) radius 2.25 projected
  circle A14 centre (-62, 278.7903) radius 2.1 projected
  line L4 (-40.5034, 109.2111) -> (-95.4966, 109.2111) projected
  arc A15 (-99.3012, 117.4553) -> (-95.4966, 109.2111) centre (-95.4966, 114.2111) ccw projected
  line L5 (-99.3012, 117.4553) -> (-71.8046, 149.7017) projected
  arc A16 (-64.1954, 149.7017) -> (-71.8046, 149.7017) centre (-68, 146.4575) ccw projected
  line L6 (-64.1954, 149.7017) -> (-36.6988, 117.4553) projected
  arc A17 (-40.5034, 109.2111) -> (-36.6988, 117.4553) centre (-40.5034, 114.2111) ccw projected
  arc A18 (-118, 139.9204) -> (-109.1954, 136.6761) centre (-113, 139.9204) ccw projected
  line L7 (-118, 139.9204) -> (-118, 199.2309) projected
  arc A19 (-109.1954, 202.4751) -> (-118, 199.2309) centre (-113, 199.2309) ccw projected
  line L8 (-109.1954, 202.4751) -> (-83.9083, 172.8198) projected
  arc A20 (-83.9083, 166.3314) -> (-83.9083, 172.8198) centre (-87.7129, 169.5756) ccw projected
  line L9 (-83.9083, 166.3314) -> (-109.1954, 136.6761) projected
  circle A21 centre (-19, 278.7903) radius 2.1 projected
  circle A22 centre (-46.8597, 40.7124) radius 5.5 projected
  arc A23 (-18, 199.2309) -> (-26.8046, 202.4751) centre (-23, 199.2309) ccw projected
  line L10 (-18, 199.2309) -> (-18, 139.9204) projected
  arc A24 (-26.8046, 136.6761) -> (-18, 139.9204) centre (-23, 139.9204) ccw projected
  line L11 (-26.8046, 136.6761) -> (-52.0917, 166.3314) projected
  arc A25 (-52.0917, 172.8198) -> (-52.0917, 166.3314) centre (-48.2871, 169.5756) ccw projected
  line L12 (-52.0917, 172.8198) -> (-26.8046, 202.4751) projected
  line L13 (0, 267.9415) -> (0, 27.3695) projected
  arc A26 (0, 267.9415) -> (-13.124, 288.8888) centre (-37, 259.345) ccw projected
  arc A27 (-13.124, 288.8888) -> (-16.2668, 290) centre (-16.2668, 285) ccw projected
  line L14 (-16.2668, 290) -> (-72.7377, 290) projected
  arc A28 (-72.7377, 290) -> (-74.4347, 289.7032) centre (-72.7377, 285) ccw projected
  arc A29 (-74.4347, 289.7032) -> (-150, 221.3595) centre (-28.8449, 163.3493) ccw projected
  line L15 (-150, 62.7066) -> (-150, 221.3595) projected
  arc A30 (-150, 62.7066) -> (-147.407, 58.3241) centre (-145, 62.7066) ccw projected
  arc A31 (-147.407, 58.3241) -> (-4.2138, 22.4317) centre (-33.7733, 208.0855) ccw projected
  arc A32 (-4.2138, 22.4317) -> (0, 27.3695) centre (-5, 27.3695) ccw projected
  line L16 (-58.75, 243.345) -> (-58.75, 263.345) projected
  arc A33 (-54.45, 263.345) -> (-58.75, 263.345) centre (-56.6, 263.345) ccw projected
  line L17 (-54.45, 263.345) -> (-54.45, 243.345) projected
  arc A34 (-58.75, 243.345) -> (-54.45, 243.345) centre (-56.6, 243.345) ccw projected
  line L18 (-23.75, 263.345) -> (-23.75, 243.345) projected
  arc A35 (-50.25, 243.345) -> (-23.75, 243.345) centre (-37, 243.345) ccw projected
  line L19 (-50.25, 243.345) -> (-50.25, 263.345) projected
  arc A36 (-23.75, 263.345) -> (-50.25, 263.345) centre (-37, 263.345) ccw projected
  line L20 (-19.55, 243.345) -> (-19.55, 263.345) projected
  arc A37 (-15.25, 263.345) -> (-19.55, 263.345) centre (-17.4, 263.345) ccw projected
  line L21 (-15.25, 263.345) -> (-15.25, 243.345) projected
  arc A38 (-19.55, 243.345) -> (-15.25, 243.345) centre (-17.4, 243.345) ccw projected
  line L22 (-86.829, 224.9401) -> (-49.171, 224.9401) projected
  arc A39 (-46.1273, 218.3448) -> (-49.171, 224.9401) centre (-49.171, 220.9401) ccw projected
  line L23 (-46.1273, 218.3448) -> (-64.9563, 196.2632) projected
  arc A40 (-71.0437, 196.2632) -> (-64.9563, 196.2632) centre (-68, 198.8586) ccw projected
  line L24 (-71.0437, 196.2632) -> (-89.8727, 218.3448) projected
  arc A41 (-86.829, 224.9401) -> (-89.8727, 218.3448) centre (-86.829, 220.9401) ccw projected
  line L25 (-59.5472, 66.9978) -> (-59.5472, 50.6)
  arc A42 (-83.5472, 50.6) -> (-59.5472, 50.6) centre (-71.5472, 50.6) ccw
  line L26 (-83.5472, 50.6) -> (-83.5472, 66.9978)
  arc A43 (-59.5472, 66.9978) -> (-83.5472, 66.9978) centre (-71.5472, 66.9978) ccw
  line L27 (-53.9492, 66.9978) -> (-53.9492, 50.0917)
  arc A44 (-57.1492, 50.0917) -> (-53.9492, 50.0917) centre (-55.5492, 50.0917) ccw
  line L28 (-57.1492, 50.0917) -> (-57.1492, 66.9978)
  arc A45 (-53.9492, 66.9978) -> (-57.1492, 66.9978) centre (-55.5492, 66.9978) ccw
  line L29 (-71.5472, 50.6) -> (-71.5472, 66.9978)
  circle A46 centre (-37, 253.345) radius 13.25 projected
  circle A47 centre (-17.4, 253.345) radius 2.15 projected
  circle A48 centre (-56.6, 253.345) radius 2.15 projected
  line L30 (-26.8046, 136.6761) -> (-52.0917, 166.3314) projected
  arc A49 (-52.0917, 172.8198) -> (-52.0917, 166.3314) centre (-48.2871, 169.5756) ccw projected
  line L31 (-52.0917, 172.8198) -> (-26.8046, 202.4751) projected
  arc A50 (-18, 199.2309) -> (-26.8046, 202.4751) centre (-23, 199.2309) ccw projected
  line L32 (-18, 199.2309) -> (-18, 139.9204) projected
  arc A51 (-26.8046, 136.6761) -> (-18, 139.9204) centre (-23, 139.9204) ccw projected
  line L33 (-109.1954, 202.4751) -> (-83.9083, 172.8198) projected
  arc A52 (-83.9083, 166.3314) -> (-83.9083, 172.8198) centre (-87.7129, 169.5756) ccw projected
  line L34 (-83.9083, 166.3314) -> (-109.1954, 136.6761) projected
  arc A53 (-118, 139.9204) -> (-109.1954, 136.6761) centre (-113, 139.9204) ccw projected
  line L35 (-118, 139.9204) -> (-118, 199.2309) projected
  arc A54 (-109.1954, 202.4751) -> (-118, 199.2309) centre (-113, 199.2309) ccw projected
  line L36 (-36.6988, 221.6959) -> (-64.1954, 189.4495) projected
  arc A55 (-71.8046, 189.4495) -> (-64.1954, 189.4495) centre (-68, 192.6937) ccw projected
  line L37 (-71.8046, 189.4495) -> (-99.3012, 221.6959) projected
  arc A56 (-95.4966, 229.9401) -> (-99.3012, 221.6959) centre (-95.4966, 224.9401) ccw projected
  line L38 (-95.4966, 229.9401) -> (-40.5034, 229.9401) projected
  arc A57 (-36.6988, 221.6959) -> (-40.5034, 229.9401) centre (-40.5034, 224.9401) ccw projected
  line L39 (-99.3012, 117.4553) -> (-71.8046, 149.7017) projected
  arc A58 (-64.1954, 149.7017) -> (-71.8046, 149.7017) centre (-68, 146.4575) ccw projected
  line L40 (-64.1954, 149.7017) -> (-36.6988, 117.4553) projected
  arc A59 (-40.5034, 109.2111) -> (-36.6988, 117.4553) centre (-40.5034, 114.2111) ccw projected
  line L41 (-40.5034, 109.2111) -> (-95.4966, 109.2111) projected
  arc A60 (-99.3012, 117.4553) -> (-95.4966, 109.2111) centre (-95.4966, 114.2111) ccw projected
  arc A61 (-4.2138, 22.4317) -> (0, 27.3695) centre (-5, 27.3695) ccw projected
  line L42 (0, 267.9415) -> (0, 27.3695) projected
  arc A62 (0, 267.9415) -> (-13.124, 288.8888) centre (-37, 259.345) ccw projected
  arc A63 (-13.124, 288.8888) -> (-16.2668, 290) centre (-16.2668, 285) ccw projected
  line L43 (-16.2668, 290) -> (-72.7377, 290) projected
  arc A64 (-72.7377, 290) -> (-74.4347, 289.7032) centre (-72.7377, 285) ccw projected
  arc A65 (-74.4347, 289.7032) -> (-150, 221.3595) centre (-28.8449, 163.3493) ccw projected
  line L44 (-150, 62.7066) -> (-150, 221.3595) projected
  arc A66 (-150, 62.7066) -> (-147.5924, 58.4311) centre (-145, 62.7066) ccw projected
  arc A67 (-147.1688, 58.1436) -> (-147.5924, 58.4311) centre (-150.1848, 54.1556) ccw projected
  arc A68 (-147.1688, 58.1436) -> (-4.2138, 22.4317) centre (-33.7733, 208.0855) ccw projected
  circle A69 centre (-27.8653, 29.2915) radius 2.1 projected
  circle A70 centre (-62, 278.7903) radius 2.1 projected
  circle A71 centre (-19, 278.7903) radius 2.1 projected
  circle A72 centre (-46.8597, 40.7124) radius 5.5 projected
  circle A73 centre (-8, 239.9401) radius 2.25 projected
  circle A74 centre (-8, 169.5272) radius 2.25 projected
  circle A75 centre (-8, 99.2111) radius 2.25 projected
  circle A76 centre (-81, 273) radius 5.5 projected
  circle A77 centre (-115, 59.0909) radius 5.5 projected
  circle A78 centre (-94.3579, 89.0409) radius 2.25 projected
  circle A79 centre (-87.5451, 59.053) radius 1.6 projected
  circle A80 centre (-55.5492, 58.5447) radius 1.6 projected
  circle A81 centre (-63.3281, 72.5265) radius 1.6 projected
  circle A82 centre (-71.5472, 58.7989) radius 12 projected
  circle A83 centre (-142.3579, 79.1409) radius 2.25 projected
  circle A84 centre (-94.3579, 79.1409) radius 2.25 projected
  circle A85 centre (-79.7662, 45.0713) radius 1.6 projected
  circle A86 centre (-63.7683, 44.8172) radius 1.6 projected
  circle A87 centre (-79.3261, 72.7806) radius 1.6 projected
  circle A88 centre (-142.3579, 89.0409) radius 2.25 projected
  point P0 (0, 0)
  point P1 (-34.0897, 48.1931)
  point P2 (-71.5472, 58.7989)
  point P3 (-50.25, 253.345)
  point P4 (-23.75, 253.345)
  constraints: 18 end point, 16 point on circle, 8 centre point, 1 midpoint, 1 vertical
extrude "Выдавливание14" cut sketch "Эскиз16" against normal blind 10 contours A79 A6 A8 | L0 A5 L1 A79 | A79 L2 A7 L3 | L16 A48 L17 A34 | L16 A33 L17 A48 | A48 | L18 A46 L19 A36 | L18 A35 L19 A46 | L20 A47 L21 A38 | L20 A37 L21 A47 | A47 | L25 A82 L26 A43 | A82 | L25 A42 L26 A82 | L27 A80 L28 A45 | A80 | L27 A44 L28 A80 | A85 | A86
extrude "Выдавливание15" add sketch "Эскиз16" against normal up to surface (4 mm away) contours L36 A55 L37 A56 L38 A57